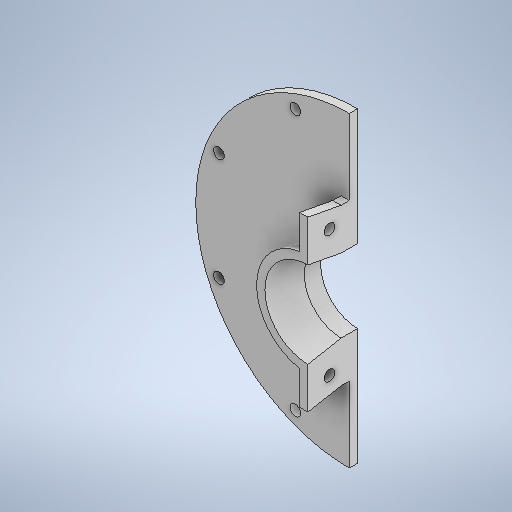
# Autodesk Inventor part: rohr-mount-v2
Saved by Autodesk Inventor 2025 (Build 290162000, 162)
## iProperties
Created: 2024-04-18
Part Number: rohr-mount-v2
Material: Generisch
Document SubType Name: Modeling
Designer: nst
Density: 1 g/cm^3
Appearance: Vorgabe
Author: nst
Autodesk Inventor part; units mm, degrees
ref_plane "YZ Plane" through (0, 0, 0) normal (1, 0, 0) x (0, 1, 0)
ref_plane "XZ Plane" through (0, 0, 0) normal (0, 1, 0) x (-1, 0, 0)
ref_plane "XY Plane" through (0, 0, 0) normal (0, 0, 1) x (1, 0, 0)
sketch "Skizze1" plane through (0, 0, 0) normal (0, 1, 0) x (-1, 0, 0)
  circle A0 centre (0, 0) radius 22.25
  circle A1 centre (0, 0) radius 27.25
  line L0 (5, 47.25) -> (-5, 47.25)
  line L1 (-5, 47.25) -> (-5, -47.25)
  line L2 (-5, -47.25) -> (5, -47.25)
  line L3 (5, -47.25) -> (5, 47.25)
  line L4 (5, 47.25) -> (-5, -47.25) construction
  line L5 (-5, 47.25) -> (5, -47.25) construction
  line L6 (0, 47.25) -> (0, -47.25)
  point P0 (0, 22.25)
  point P1 (0, -22.25)
  point P2 (5, -26.7874)
  point P3 (5, 26.7874)
  dimension "d0" = 44.5
  dimension "d1" = 54.5
  dimension "d2" = 10
  dimension "d3" = 94.5
  constraints: 14 end point, 4 midpoint, 2 centre point, 2 coincident, 2 parallel, 1 horizontal, 1 perpendicular
  measures "d0" diameter of A0
  measures "d1" diameter of A1
  measures "d2" distance of L2.end L1.end
  measures "d3" distance of L1.end L0.end
extrude "Extrusion1" add sketch "Skizze1" along normal blind 5 contours A0 L3 A1 | A0 L6 A1 L3 | L3 A1 L6 A0 | A1 L6 L0 L3 | L3 L2 L6 A1
sketch "Skizze4" plane through (0, 5, 0) normal (0, 1, 0) x (1, 0, 0)
  circle A0 centre (0, 0) radius 22.25
  circle A1 centre (0, 0) radius 92.8
  circle A2 centre (0, 0) radius 72.8
  line L0 (0, -92.8) -> (0, 92.8)
  point P0 (0, 22.25)
  point P1 (0, -22.25)
  dimension "d23" = 185.6
  dimension "d24" = 145.6
  dimension "d43" = 44.5
  constraints: 3 centre point, 3 coincident, 2 end point, 2 point on circle, 1 vertical
  measures "d23" diameter of A1
  measures "d24" diameter of A2
  measures "d43" diameter of A0
extrude "Extrusion4" add sketch "Skizze4" along normal blind 5 contours A0 L0 A2 | A2 L0 A1 picked at (-55.7302, 0.894) picked at (-74.476, -42.8466)
sketch "Skizze5" plane through (0, 10, 0) normal (0, 1, 0) x (1, 0, 0)
  circle A0 centre (0, 0) radius 52.8
  arc A1 (0, 92.8) -> (0, -92.8) centre (0, 0) ccw projected
  line L0 (0, 0) -> (72.8, 0) construction
  line L1 (0, 0) -> (72.8, 0) construction
  circle A2 centre (0, 0) radius 85.3
  line L2 (0, 0) -> (-35.513, 85.736)
  line L3 (0, 0) -> (92.8, 0) construction
  line L4 (0, 0) -> (-85.736, 35.513)
  line L5 (0, 0) -> (92.8, 0) construction
  line L6 (0, 0) -> (-35.513, -85.736)
  line L7 (0, 0) -> (92.8, 0) construction
  line L8 (0, 0) -> (-85.736, -35.513)
  line L9 (0, 0) -> (92.8, 0) construction
  circle A3 centre (-32.6429, -78.8069) radius 3.25
  circle A4 centre (-78.8069, -32.6429) radius 3.25
  circle A5 centre (-78.8069, 32.6429) radius 3.25
  circle A6 centre (-32.6429, 78.8069) radius 3.25
  circle A7 centre (0, 0) radius 77.8
  dimension "d27" = 105.6
  dimension "d31" = 170.6
  dimension "d32" = 112.5
  dimension "d33" = 157.5
  dimension "d34" = 112.5
  dimension "d35" = 157.5
  dimension "d36" = 6.5
  dimension "d37" = 6.5
  dimension "d38" = 6.5
  dimension "d39" = 6.5
  dimension "d42" = 155.6
  constraints: 20 end point, 8 point on circle, 7 centre point, 6 horizontal, 4 equal length, 4 point on line, 3 coincident
  measures "d27" diameter of A0
  measures "d31" diameter of A2
  measures "d32" angle of L3 L2
  measures "d33" angle of L5 L4
  measures "d34" angle of L6 L7
  measures "d35" angle of L8 L9
  measures "d36" diameter of A3
  measures "d37" diameter of A4
  measures "d38" diameter of A5
  measures "d39" diameter of A6
  measures "d42" diameter of A7
extrude "Extrusion5" cut sketch "Skizze5" against normal through all contours A6 A2 L2 | L2 A2 A6 | A3 A2 L6 | L6 A2 A3 | A5 A2 L4 | L4 A2 A5 | L2 A6 A2 | A2 A6 L2 | A4 A2 L8 | L8 A2 A4 | L6 A3 A2 | A2 A3 L6 | L4 A5 A2 | A2 A5 L4 | L8 A4 A2 | A2 A4 L8
sketch "Skizze6" plane through (0, 0, 0) normal (0, -1, 0) x (1, 0, 0)
  circle A0 centre (0, 0) radius 38.25
  line L0 (5, 63.25) -> (-5, 63.25)
  line L1 (-5, 63.25) -> (-5, -63.25)
  line L2 (-5, -63.25) -> (5, -63.25)
  line L3 (5, -63.25) -> (5, 63.25)
  line L4 (5, 63.25) -> (-5, -63.25) construction
  line L5 (-5, 63.25) -> (5, -63.25) construction
  circle A1 centre (0, 0) radius 43.25
  circle A2 centre (0, 0) radius 22.25
  line L6 (0, -47.25) -> (0, -92.8) projected
  line L7 (0, -63.25) -> (0, 63.25)
  point P0 (-5, 42.96)
  point P1 (-5, -42.96)
  point P2 (0, -22.25)
  point P3 (0, 22.25)
  dimension "d44" = 76.5
  dimension "d45" = 10
  dimension "d46" = 126.5
  dimension "d47" = 86.5
  constraints: 14 end point, 4 midpoint, 3 centre point, 3 coincident, 2 parallel, 1 horizontal, 1 perpendicular, 1 point on line
  measures "d44" diameter of A0
  measures "d45" distance of L2.end L1.end
  measures "d46" distance of L1.end L0.end
  measures "d47" diameter of A1
extrude "Extrusion6" add sketch "Skizze6" along normal blind 85 contours L7 A2 L1 A0 | A0 L1 A1 L7 | L7 A1 L1 A0 | A0 L1 A2 L7 | L1 A2 A0 | A0 L1 A1 | A1 L1 L0 L7 | L7 L6 L2 L1 A1
chamfer "Fasen1" distance 16 distance2 85 1 edges at (-22.25, -85, 0) measured on face at (-1.6667, -85, -42.82)
chamfer "Fasen2" distance 85 angle 10.66 1 edges at (-2.5, 0, -63.25) measured on face at (-3.3333, -28.3333, -63.25)
chamfer "Fasen3" distance 85 distance2 16 1 edges at (-2.5, 0, 63.25) measured on face at (-1.6667, -28.3333, 63.25)
chamfer "Fasen4" distance 85 distance2 16 1 edges at (-43.25, 0, 0) measured on face at (-38.2627, -56.6667, -20.1626)
sketch "Skizze7" plane through (0, -85, 0) normal (0, -1, 0) x (1, 0, 0)
  circle A0 centre (0, 0) radius 65
  dimension "d62" = 130
  constraints: 1 centre point, 1 coincident
  measures "d62" diameter of A0
extrude "Extrusion7" cut sketch "Skizze7" against normal blind 65
sketch "Skizze8" plane through (-5, 5, -47.25) normal (-1, 0, 0) x (0, 0, 1)
  circle A0 centre (9, -12) radius 3.25
  line L0 (-3.7651, -25) -> (16.641, -25) projected
  line L1 (0, -5) -> (0, 0) projected
  point P0 (47.25, -5)
  dimension "d65" = 6.5
  dimension "d66" = 13
  dimension "d67" = 9
  constraints: 1 centre point
  measures "d65" diameter of A0
  measures "d66" distance from line of A0.centre L0
  measures "d67" distance from line of A0.centre L1
sketch "Skizze9" plane through (-5, 5, 26.7874) normal (-1, 0, 0) x (0, 0, 1)
  circle A0 centre (11.4626, -12) radius 3.25
  line L0 (3.8217, -25) -> (24.2273, -25) projected
  line L1 (20.4626, -5) -> (20.4626, 0) projected
  point P0 (-26.7874, -5)
  dimension "d68" = 6.5
  dimension "d69" = 13
  dimension "d70" = 9
  constraints: 1 centre point
  measures "d68" diameter of A0
  measures "d69" distance from line of L0 A0.centre
  measures "d70" distance from line of A0.centre L1
extrude "Extrusion8" cut sketch "Skizze8" against normal through all
extrude "Extrusion9" cut sketch "Skizze9" against normal through all
